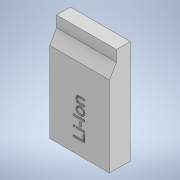
# Autodesk Inventor part: Li-IonBattery
Saved by Autodesk Inventor 2020 (Build 240168000, 168)
## iProperties
Created: 2020-04-08
Part Number: Li-IonBattery
Material: Generic
Document SubType Name: Modeling
Designer: Samuele
Density: 1 g/cm^3
Appearance: Default
Author: Samuele
Autodesk Inventor part; units mm, degrees
ref_plane "YZ Plane" through (0, 0, 0) normal (1, 0, 0) x (0, 1, 0)
ref_plane "XZ Plane" through (0, 0, 0) normal (0, 1, 0) x (-1, 0, 0)
ref_plane "XY Plane" through (0, 0, 0) normal (0, 0, 1) x (1, 0, 0)
sketch "Sketch1" plane through (0, 0, 0) normal (0, 0, 1) x (1, 0, 0)
  line L0 (0, 0) -> (26, 0)
  line L1 (26, 0) -> (26, 45)
  line L2 (26, 45) -> (0, 45)
  line L3 (0, 45) -> (0, 0)
  dimension "d0" = 26
  dimension "d1" = 45
  constraints: 8 end point, 2 parallel, 1 horizontal, 1 perpendicular
  measures "d0" distance of L2.end L1.end
  measures "d1" distance of L1.end L0.end
extrude "Extrusion1" add sketch "Sketch1" along normal blind 6
sketch "Sketch2" plane through (0, 0, 6) normal (0, 0, 1) x (1, 0, 0)
  line L0 (26, 0) -> (26, 45) projected
  line L1 (0, 0) -> (26, 0)
  line L2 (26, 0) -> (26, 35)
  line L3 (26, 35) -> (0, 35)
  line L4 (0, 35) -> (0, 0)
  dimension "d4" = 35
  constraints: 8 end point, 2 parallel, 1 horizontal, 1 perpendicular, 1 point on line
  measures "d4" distance of L2.end L1.end
extrude "Extrusion2" add sketch "Sketch2" along normal blind 3
draft "FaceDraft1" angle 60 pull direction (0, 0, 1) faces at (17.3333, 35, 7) fixed edges at (13, 35, 9)
sketch "Sketch3" plane through (0, 0, 9) normal (0, 0, 1) x (1, 0, 0)
  line L0 (10.2597, 5.4477) -> (10.2597, 19.6754) construction
  line L1 (10.2597, 19.6754) -> (17.2769, 19.6754) construction
  line L2 (17.2769, 19.6754) -> (17.2769, 5.4477) construction
  line L3 (17.2769, 5.4477) -> (10.2597, 5.4477) construction
  line L4 (0, 0) -> (26, 0) projected
  line L5 (13, 0) -> (13, 5.1104)
  line L6 (15.2597, 5.9584) -> (10.2597, 5.9584)
  line L7 (10.2597, 5.9584) -> (10.2597, 6.6215)
  line L8 (10.2597, 6.6215) -> (14.669, 6.6215)
  line L9 (14.669, 6.6215) -> (14.669, 9.0834)
  line L10 (14.669, 9.0834) -> (15.2597, 9.0834)
  line L11 (15.2597, 9.0834) -> (15.2597, 5.9584)
  line L12 (15.2597, 9.7961) -> (11.6354, 9.7961)
  line L13 (11.6354, 9.7961) -> (11.6354, 10.4096)
  line L14 (11.6354, 10.4096) -> (15.2597, 10.4096)
  line L15 (15.2597, 10.4096) -> (15.2597, 9.7961)
  line L16 (10.9647, 9.7961) -> (10.2597, 9.7961)
  line L17 (10.2597, 9.7961) -> (10.2597, 10.4096)
  line L18 (10.2597, 10.4096) -> (10.9647, 10.4096)
  line L19 (10.9647, 10.4096) -> (10.9647, 9.7961)
  line L20 (13.7581, 11.0994) -> (13.1408, 11.0994)
  line L21 (13.1408, 11.0994) -> (13.1408, 12.9897)
  line L22 (13.1408, 12.9897) -> (13.7581, 12.9897)
  line L23 (13.7581, 12.9897) -> (13.7581, 11.0994)
  line L24 (15.2597, 13.8586) -> (10.2597, 13.8586)
  line L25 (10.2597, 13.8586) -> (10.2597, 14.5217)
  line L26 (10.2597, 14.5217) -> (15.2597, 14.5217)
  line L27 (15.2597, 14.5217) -> (15.2597, 13.8586)
  spline S0 degree 2 poles (13.4456, 15.3791) (12.4433, 15.3791) (11.9593, 15.9394) knots 0 0 0 1 1 1
  spline S1 degree 2 poles (11.9593, 15.9394) (11.5554, 16.4043) (11.5554, 17.075) knots 0 0 0 1 1 1
  spline S2 degree 2 poles (11.5554, 17.075) (11.5554, 17.822) (12.5348, 18.7709) (13.3961, 18.7709) knots 0 0 0 1 2 2 2
  spline S3 degree 2 poles (13.3961, 18.7709) (14.0935, 18.7709) (14.8976, 18.3517) (15.3397, 17.5514) (15.3397, 17.075) knots 0 0 0 1 2 3 3 3
  spline S4 degree 2 poles (15.3397, 17.075) (15.3397, 16.3166) (14.3641, 15.3791) (13.4456, 15.3791) knots 0 0 0 1 2 2 2
  spline S5 degree 2 poles (13.4494, 16.0118) (14.143, 16.0118) (14.8366, 16.6177) (14.8366, 17.075) knots 0 0 0 1 2 2 2
  spline S6 degree 2 poles (14.8366, 17.075) (14.8366, 17.5323) (14.1392, 18.1383) (13.4266, 18.1383) knots 0 0 0 1 2 2 2
  spline S7 degree 2 poles (13.4266, 18.1383) (12.7558, 18.1383) (12.0622, 17.5285) (12.0622, 17.075) knots 0 0 0 1 2 2 2
  spline S8 degree 2 poles (12.0622, 17.075) (12.0622, 16.6177) (12.752, 16.0118) (13.4494, 16.0118) knots 0 0 0 1 2 2 2
  line L28 (15.2597, 19.4912) -> (11.6354, 19.4912)
  line L29 (11.6354, 19.4912) -> (11.6354, 20.0438)
  line L30 (11.6354, 20.0438) -> (12.1499, 20.0438)
  spline S9 degree 2 poles (12.1499, 20.0438) (11.5554, 20.4439) (11.5554, 21.1947) knots 0 0 0 1 1 1
  spline S10 degree 2 poles (11.5554, 21.1947) (11.5554, 21.5224) (11.7917, 22.0712) (12.1728, 22.3456) (12.4357, 22.399) knots 0 0 0 1 2 3 3 3
  spline S11 degree 2 poles (12.4357, 22.399) (12.6072, 22.4333) (13.034, 22.4333) knots 0 0 0 1 1 1
  line L31 (13.034, 22.4333) -> (15.2597, 22.4333)
  line L32 (15.2597, 22.4333) -> (15.2597, 21.8197)
  line L33 (15.2597, 21.8197) -> (13.0569, 21.8197)
  spline S12 degree 2 poles (13.0569, 21.8197) (12.6834, 21.8197) (12.31, 21.6749) (12.0889, 21.3128) (12.0889, 21.0651) knots 0 0 0 1 2 3 3 3
  spline S13 degree 2 poles (12.0889, 21.0651) (12.0889, 20.6726) (12.5882, 20.1048) (13.2818, 20.1048) knots 0 0 0 1 2 2 2
  line L34 (13.2818, 20.1048) -> (15.2597, 20.1048)
  line L35 (15.2597, 20.1048) -> (15.2597, 19.4912)
  constraints: 2 end point, 1 midpoint, 1 vertical, 2 other
extrude "Extrusion3" cut sketch "Sketch3" against normal blind 1
body "Solid1"
